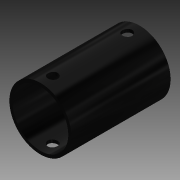
# Autodesk Inventor part: VersaRollerTestPart
Saved by Autodesk Inventor 2022 (Build 260153000, 153)
## iProperties
Created: 2021-08-05
Part Number: VersaRollerTestPart
Material: Aluminum 6061
Document SubType Name: Modeling
Designer: Max Boord
Density: 2.7 g/cm^3
Appearance: Glossy - Black
RollerLength: 2.000 in
Author: Max Boord
Autodesk Inventor part; units mm, degrees
ref_plane "YZ Plane" through (0, 0, 0) normal (1, 0, 0) x (0, 1, 0)
ref_plane "XZ Plane" through (0, 0, 0) normal (0, 1, 0) x (-1, 0, 0)
ref_plane "XY Plane" through (0, 0, 0) normal (0, 0, 1) x (1, 0, 0)
sketch "Sketch16" plane through (0, 0, 0) normal (0, 0, 1) x (1, 0, 0)
  circle A0 centre (0, 0) radius 14.2875
  circle A1 centre (0, 0) radius 15.875
  dimension "d197" = 28.575
  dimension "d198" = 31.75
  constraints: 2 centre point, 1 coincident
  measures "d197" diameter of A0
  measures "d198" diameter of A1
extrude "Extrusion1" add sketch "Sketch16" along normal mid plane 50.8
sketch "Sketch17" plane through (0, 0, 0) normal (0, 1, 0) x (-1, 0, 0)
  line L0 (-15.875, -25.4) -> (15.875, -25.4) projected
  line L1 (0, 0) -> (0, 19.05)
  circle A0 centre (0, 19.05) radius 2.4892
  line L2 (15.875, 25.4) -> (-15.875, 25.4) projected
  line L3 (-22.225, 0) -> (22.225, 0) projected
  circle A1 centre (0, -19.05) radius 2.4892
  point P0 (15.875, -25.4)
  dimension "d202" = 4.9784
  dimension "d205" = 6.35
  constraints: 2 centre point, 2 coincident, 2 end point, 2 symmetric about line, 1 vertical, 2 other
  measures "d202" diameter of A0
  measures "d205" distance from line of L2 L1.end
extrude "Extrusion2" cut sketch "Sketch17" along normal mid plane 50.8 contours A0
extrude "Extrusion3" cut sketch "Sketch17" along normal mid plane 50.8 contours A1
body "Solid1"
